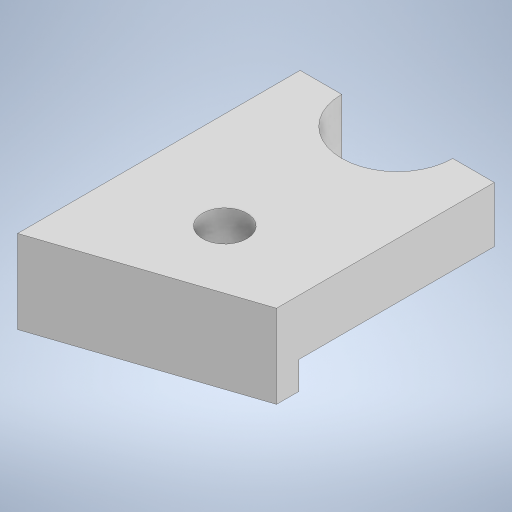
# Autodesk Inventor part: plungerholdermod1
Saved by Autodesk Inventor 2023 (Build 270158000, 158)
## iProperties
Created: 2025-09-27
Part Number: plungerholdermod1
Material: Generic
Document SubType Name: Modeling
Designer: ptato_qo49uko
Density: 1 g/cm^3
Appearance: Default
Author: ptato_qo49uko
Autodesk Inventor part; units mm, degrees
ref_plane "YZ Plane" through (0, 0, 0) normal (1, 0, 0) x (0, 1, 0)
ref_plane "XZ Plane" through (0, 0, 0) normal (0, 1, 0) x (-1, 0, 0)
ref_plane "XY Plane" through (0, 0, 0) normal (0, 0, 1) x (1, 0, 0)
sketch "Sketch1" plane through (0, 0, 0) normal (0, 1, 0) x (-1, 0, 0)
  line L0 (-9.1057, 3.648) -> (-9.1057, -9.552)
  line L1 (4.8943, -9.552) -> (4.8943, 8.308)
  line L2 (4.8943, 8.308) -> (-9.1057, 3.648)
  line L3 (-2.1057, 5.978) -> (-2.1057, 1.978)
  circle A0 centre (-2.1057, 0.378) radius 1.6
  line L4 (4.8943, -9.552) -> (4.8943, -12.052)
  line L5 (-9.1057, -9.552) -> (-9.1057, -12.052)
  line L6 (4.8943, -12.052) -> (-9.1057, -12.052)
  circle A1 centre (-2.1057, -12.052) radius 4
  line L7 (-2.1057, -1.222) -> (-2.1057, -8.052)
  line L8 (4.8943, 1.978) -> (-2.1057, 1.978)
  line L9 (-9.1057, 1.978) -> (-2.1057, 1.978)
  point P0 (0, 0)
  point P1 (1.8943, -12.052)
  point P2 (-6.1057, -12.052)
  dimension "d8" = 3.2
  dimension "d19" = 8
  dimension "d5" = 13.2
  dimension "d6" = 4
  dimension "d10" = 17.86
  dimension "d13" = 14
  dimension "d16" = 2.5
  constraints: 20 end point, 4 vertical, 3 point on line, 2 horizontal, 2 midpoint, 2 perpendicular, 1 parallel, 1 vertical alignment, 5 other
  measures "d5" distance of L0.start L0.end
  measures "d6" distance of L3.start L3.end
  measures "d10" distance of L1.start L1.end
  measures "d13" distance of L0.end L1.start
  measures "d16" distance of L1.start L4.end
extrude "Extrusion2" add sketch "Sketch1" along normal blind 4 contours L2 L3 L9 L0 | L9 A0 L7 A1 L6 L5 L0 | L2 L1 L8 L3 | L8 L1 L4 L6 A1 L7 A0
sketch "Sketch2" plane through (0, 0, 0) normal (0, -1, 0) x (1, 0, 0)
  line L0 (9.1057, 3.648) -> (9.1057, -12.052) projected
  line L1 (9.1057, 2.0387) -> (-4.8943, 2.0387)
  line L2 (-4.8943, -12.052) -> (-4.8943, 8.308) projected
  line L3 (-4.8943, 2.0387) -> (-4.8943, 8.308)
  line L4 (-4.8943, 8.308) -> (9.1057, 3.648) projected
  line L5 (-4.8943, 8.308) -> (9.1057, 3.648)
  line L6 (9.1057, 3.648) -> (9.1057, 2.0387)
  point P0 (0, 0)
  constraints: 8 end point, 3 collinear, 1 perpendicular, 1 point on line
extrude "Extrusion3" add sketch "Sketch2" along normal blind 2
body "Solid2"
